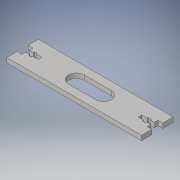
# Autodesk Inventor part: A8-0006
Saved by Autodesk Inventor 2016 SP2 (Build 200236200, 236)
## iProperties
Created: 2017-04-22
Part Number: A8-0006
Material: Generic
Document SubType Name: Modeling
Designer: EV
Density: 1 g/cm^3
Appearance: Default
Author: EV
Autodesk Inventor part; units mm, degrees
ref_plane "YZ Plane" through (0, 0, 0) normal (1, 0, 0) x (0, 1, 0)
sketch "Sketch1" plane through (0, 0, 0) normal (0, 1, 0) x (-1, 0, 0)
  line L0 (64, 0) -> (-64, 0)
  line L1 (-64, 0) -> (-64, -30)
  line L2 (-64, -30) -> (64, -30)
  line L3 (64, -30) -> (64, 0)
  line L4 (13, -15) -> (-13, -15) construction
  line L5 (13, -7.5) -> (-13, -7.5)
  line L6 (-13, -22.5) -> (13, -22.5)
  arc A0 (13, -22.5) -> (13, -7.5) centre (13, -15) ccw
  arc A1 (-13, -7.5) -> (-13, -22.5) centre (-13, -15) ccw
  line L7 (13, -15) -> (64, -15) construction
  line L8 (0, -15) -> (0, -30) construction
  point P0 (0, 0)
  point P1 (0, 0)
  dimension "d0" = 128
  dimension "d1" = 30
  dimension "d2" = 15
  dimension "d3" = 26
  constraints: 20 end point, 4 midpoint, 4 point on circle, 4 tangent, 3 parallel, 3 perpendicular, 2 centre point, 2 horizontal, 1 coincident
  measures "d0" distance of L0.start L0.end
  measures "d1" distance of L2.end L0.start
  measures "d2" distance between parallel lines of L6 L5
  measures "d3" distance of L4.start L4.end
extrude "Extrusion1" add sketch "Sketch1" along normal blind 4.5
sketch "Sketch2" plane through (0, 4.5, 0) normal (0, 1, 0) x (1, 0, 0)
  arc A0 (-13, 22.5) -> (-13, 7.5) centre (-13, 15) ccw construction
  line L0 (-13, 22.5) -> (13, 22.5) construction
  arc A1 (13, 7.5) -> (13, 22.5) centre (13, 15) ccw construction
  line L1 (13, 7.5) -> (-13, 7.5) construction
  line L2 (-64, 0) -> (64, 0) construction
  line L3 (64, 0) -> (64, 30) construction
  line L4 (64, 30) -> (-64, 30) construction
  line L5 (-64, 30) -> (-64, 0) construction
  line L6 (-64, 20.25) -> (-59.5, 20.25)
  line L7 (-59.5, 20.25) -> (-59.5, 16.75)
  line L8 (-59.5, 16.75) -> (-55.5, 16.75)
  line L9 (-55.5, 16.75) -> (-55.5, 18)
  line L10 (-55.5, 18) -> (-52.5, 18)
  line L11 (-52.5, 18) -> (-52.5, 16.75)
  line L12 (-52.5, 16.75) -> (-47.5, 16.75)
  line L13 (-47.5, 16.75) -> (-47.5, 13.25)
  line L14 (-47.5, 13.25) -> (-52.5, 13.25)
  line L15 (-52.5, 13.25) -> (-52.5, 12)
  line L16 (-52.5, 12) -> (-55.5, 12)
  line L17 (-55.5, 12) -> (-55.5, 13.25)
  line L18 (-55.5, 13.25) -> (-59.5, 13.25)
  line L19 (-59.5, 9.75) -> (-64, 9.75)
  line L20 (-59.5, 9.75) -> (-59.5, 13.25)
  line L21 (-64, 15) -> (-47.5, 15) construction
  line L22 (-64, 20.25) -> (-64, 9.75)
  line L23 (-64, 30) -> (-64, 0) projected
  dimension "d6" = 10.5
  dimension "d7" = 4
  dimension "d8" = 3
  dimension "d9" = 5
  dimension "d10" = 3.5
  dimension "d11" = 6
  dimension "d12" = 4.5
  constraints: 34 end point, 12 perpendicular, 10 point on line, 3 equal length, 2 midpoint, 1 collinear, 1 horizontal
  measures "d6" distance between parallel lines of L19 L6
  measures "d7" distance of L7.end L8.end
  measures "d8" distance of L9.end L10.end
  measures "d9" distance of L11.end L12.end
  measures "d10" distance between parallel lines of L18 L8
  measures "d11" distance between parallel lines of L10 L16
  measures "d12" distance of L19.start L19.end
extrude "Extrusion2" cut sketch "Sketch2" against normal through all
mirror "Mirror1" about plane through (0, 0, 0) normal (1, 0, 0) of "Extrusion2"
ref_plane "Work Plane1" through (-13, 0, -15) normal (0, 0, 1) x (1, 0, 0)
ref_plane "Work Plane2" through (0, 2.25, 0) normal (0, 1, 0) x (-1, 0, 0)
equation "\"d16\" = 0.5 * THICKNESS"
equation "\"THICKNESS\" = 4.5"
body "Solid1"
